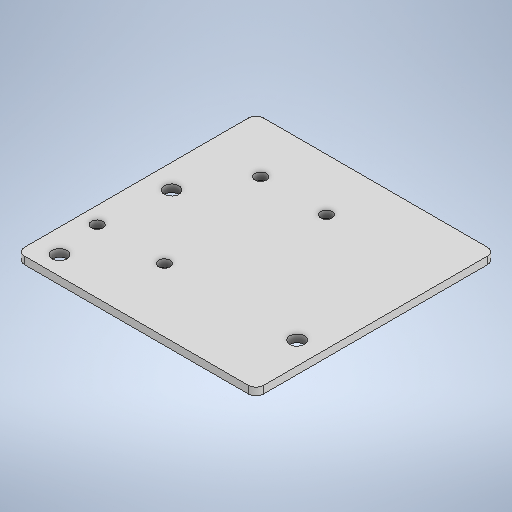
# Autodesk Inventor part: Nissan_Moter_Mount_Passenger
Saved by Autodesk Inventor 2025.1 (Build 291241000, 241)
## iProperties
Created: 2025-02-12
Part Number: Nissan_Moter_Mount_Passenger
Material: Generic
Document SubType Name: Modeling
Designer: robotics
Density: 1 g/cm^3
Appearance: Default
Author: robotics
Autodesk Inventor part; units mm, degrees
ref_plane "YZ Plane" through (0, 0, 0) normal (1, 0, 0) x (0, 1, 0)
ref_plane "XZ Plane" through (0, 0, 0) normal (0, 1, 0) x (-1, 0, 0)
ref_plane "XY Plane" through (0, 0, 0) normal (0, 0, 1) x (1, 0, 0)
sketch "Sketch1" plane through (0, 0, 0) normal (0, 1, 0) x (-1, 0, 0)
  line L0 (101.6, 101.6) -> (-101.6, 101.6)
  line L1 (-101.6, 101.6) -> (-101.6, -101.6)
  line L2 (-101.6, -101.6) -> (101.6, -101.6)
  line L3 (101.6, -101.6) -> (101.6, 101.6)
  circle A0 centre (81.28, 85.725) radius 6.35
  circle A1 centre (81.28, -9.525) radius 6.35
  circle A2 centre (-82.55, 47.625) radius 6.35
  circle A3 centre (53.1707, -57.15) radius 4.953
  circle A4 centre (-2.7093, -57.15) radius 4.953
  circle A5 centre (87.376, 47.625) radius 4.953
  circle A6 centre (30.226, 47.625) radius 4.953
  point P0 (0, 0)
  dimension "d0" = 203.2
  dimension "d1" = 203.2
  dimension "d2" = 12.7
  dimension "d3" = 15.875
  dimension "d4" = 20.32
  dimension "d6" = 95.25
  dimension "d7" = 12.7
  dimension "d8" = 19.05
  dimension "d9" = 53.975
  dimension "d10" = 9.906
  dimension "d11" = 44.45
  dimension "d12" = 55.88
  dimension "d13" = 9.906
  dimension "d14" = 9.906
  dimension "d15" = 14.224
  dimension "d16" = 9.906
  dimension "d17" = 57.15
  constraints: 8 end point, 7 centre point, 2 parallel, 1 horizontal, 1 perpendicular
  measures "d0" distance of L2.end L0.start
  measures "d1" distance of L1.end L2.end
  measures "d2" diameter of A0
  measures "d3" distance from line of L0 A0.centre
  measures "d4" distance from line of L3 A0.centre
  measures "d6" distance of A1.centre A0.centre
  measures "d7" diameter of A2
  measures "d8" distance from line of L1 A2.centre
  measures "d9" distance from line of L0 A2.centre
  measures "d10" diameter of A3
  measures "d11" distance from line of L2 A3.centre
  measures "d12" distance of A3.centre A4.centre
  measures "d13" diameter of A4
  measures "d14" diameter of A5
  measures "d15" distance from line of L3 A5.centre
  measures "d16" diameter of A6
  measures "d17" distance of A6.centre A5.centre
extrude "Extrusion1" add sketch "Sketch1" along normal blind 6.35
fillet "Fillet1" radius 6.35 4 edges at (-101.6, 3.175, 101.6) (101.6, 3.175, 101.6) (101.6, 3.175, -101.6) (-101.6, 3.175, -101.6)
body "Solid1"
